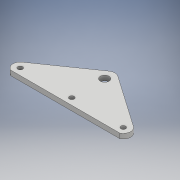
# Autodesk Inventor part: Corpo_Suporte_3_Cabos
Saved by Autodesk Inventor 2018 (Build 220112000, 112)
## iProperties
Created: 2021-08-02
Part Number: Corpo_Suporte_3_Cabos
Material: Generic
Document SubType Name: Modeling
Designer: L08619
Density: 1 g/cm^3
Appearance: Default
Author: L08619
Autodesk Inventor part; units mm, degrees
ref_plane "YZ Plane" through (0, 0, 0) normal (1, 0, 0) x (0, 1, 0)
ref_plane "XZ Plane" through (0, 0, 0) normal (0, 1, 0) x (-1, 0, 0)
ref_plane "XY Plane" through (0, 0, 0) normal (0, 0, 1) x (1, 0, 0)
sketch "Sketch1" plane through (0, 0, 0) normal (0, 0, 1) x (1, 0, 0)
  circle A0 centre (0, 0) radius 20
  circle A1 centre (-235, -150) radius 11
  circle A2 centre (0, -150) radius 11
  line L0 (-248.9435, -180) -> (0, -180)
  arc A3 (-254.009, -122.9246) -> (-248.9435, -180) centre (-235, -150) ccw
  line L1 (-254.009, -122.9246) -> (-20, 40)
  line L2 (-20, 40) -> (-10, 46.2314) construction
  spline S0 degree 2 poles (-20, 40) (-10, 46.2314) (0, 46.2314) knots 1 1 1 1.5 1.5 1.5
  line L3 (0, 87.1559) -> (0, -290.9336) construction
  line L4 (-10, 46.2314) -> (0, 46.2314) construction
  circle A4 centre (235, -150) radius 11
  line L5 (248.9435, -180) -> (0, -180)
  arc A5 (248.9435, -180) -> (254.009, -122.9246) centre (235, -150) ccw
  line L6 (254.009, -122.9246) -> (20, 40)
  line L7 (20, 40) -> (10, 46.2314) construction
  spline S1 degree 2 poles (20, 40) (10, 46.2314) (0, 46.2314) knots 1 1 1 1.5 1.5 1.5
  line L8 (10, 46.2314) -> (0, 46.2314) construction
  dimension "d0" = 40
  dimension "d1" = 22
  dimension "d3" = 22
  dimension "d4" = 150
  dimension "d5" = 30
  dimension "d8" = 235
  dimension "d9" = 40
  dimension "d12" = 120
  constraints: 10 end point, 6 centre point, 6 symmetric about line, 4 point on circle, 3 coincident, 2 point on line, 1 horizontal, 1 horizontal alignment, 1 vertical, 1 vertical alignment, 8 other
  measures "d0" diameter of A0
  measures "d1" diameter of A2
  measures "d3" diameter of A1
  measures "d4" distance of point (0, 0) A2.centre
  measures "d5" distance from line of L0 A1.centre
  measures "d8" distance of A2.centre A1.centre
  measures "d9" vertical distance of L1.end point (0, 0)
extrude "Extrusion1" add sketch "Sketch1" along normal mid plane 22.22
equation "\"d1\" = d3"
body "Solid1"
